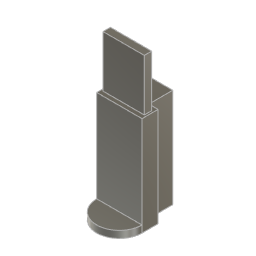
filament holder extender v1 (Autodesk Fusion 360 design; units mm, degrees)
Autodesk Fusion 360 part; units mm, degrees
note: some values were not read from the file. Set by a fixed rule: which sketch regions a step uses.
sketch "Sketch1" plane through (0, 0, 0) normal (0, 0, 1) x (1, 0, 0)
  line L0 (0, 0) -> (12.6, 0)
  line L1 (12.6, 0) -> (12.6, 13)
  line L2 (12.6, 13) -> (0, 13)
  line L3 (0, 13) -> (0, 0)
  line L4 (6.3, 0) -> (6.3, 25)
  line L5 (12.6, 13) -> (17.6, 13)
  line L6 (17.6, 13) -> (17.6, 19.7)
  line L7 (17.6, 19.7) -> (12.6, 19.7)
  line L8 (12.6, 19.7) -> (12.6, 13)
  line L9 (0, 19.7) -> (0, 13)
  line L10 (-5, 19.7) -> (0, 19.7)
  line L11 (-5, 13) -> (-5, 19.7)
  line L12 (0, 13) -> (-5, 13)
  line L13 (12.6, 19.7) -> (0, 19.7)
  line L14 (0, 19.7) -> (12.6, 13) construction
  line L15 (17.5, 18.35) -> (-4.9, 18.35)
  line L16 (-4.9, 18.35) -> (-4.9, 14.35)
  line L17 (-4.9, 14.35) -> (17.5, 14.35)
  line L18 (17.5, 14.35) -> (17.5, 18.35)
  line L19 (17.5, 18.35) -> (-4.9, 14.35) construction
  line L20 (-4.9, 18.35) -> (17.5, 14.35) construction
  line L21 (12.6, 20.7) -> (0, 20.7)
  line L22 (-6, 20.7) -> (0, 20.7)
  line L23 (-6, 12) -> (-6, 20.7)
  line L24 (-1, 12) -> (-6, 12)
  line L25 (-1, 12) -> (-1, -1)
  line L26 (-1, -1) -> (13.6, -1)
  line L27 (13.6, -1) -> (13.6, 12)
  line L28 (13.6, 12) -> (18.6, 12)
  line L29 (18.6, 12) -> (18.6, 20.7)
  line L30 (18.6, 20.7) -> (12.6, 20.7)
  point P0 (6.3, 16.35)
  dimension "d1" = 12.6
  dimension "d2" = 13
  dimension "d3" = 5
  dimension "d4" = 6.7
  dimension "d5" = 22.4
  dimension "d6" = 4
  dimension "d7" = 1
  constraint horizontal L0
  constraint vertical L1
  constraint horizontal L2
  constraint vertical L3
  constraint coincident L0.start L3.end
  constraint midpoint L0 L4.start
  constraint perpendicular L2 L4
  constraint horizontal L5
  constraint vertical L6
  constraint horizontal L7
  constraint vertical L8
  constraint symmetric L1.end L4 L2.end
  constraint symmetric L4 L5.end L11.start
  constraint symmetric L4 L6.end L10.start
  constraint symmetric L4 L7.end L9.start
  constraint horizontal L15
  constraint perpendicular L15 L16
  constraint parallel L15 L17
  constraint parallel L16 L18
  constraint coincident L19 P0
  constraint coincident L20 P0
  constraint midpoint L14 P0
  measures "d1" distance of L0.start L0.end
  measures "d2" distance of L0.start L2.end
  measures "d3" distance of L1.end L5.end
  measures "d4" distance of L1.end L7.end
  measures "d5" distance of L16.end L17.end
  measures "d6" distance of L15.end L16.end
extrude "Extrude1" add sketch "Sketch1" along normal blind 50 contours L0 L2 L3 L4 | L0 L1 L2 L4 | L2 L4 L9 L17 | L9 L10 L11 L12 L15 L16 L17 | L2 L4 L8 L17 | L9 L15 L16 L17 | L4 L9 L15 L17 | L5 L6 L7 L8 L15 L17 L18 | L4 L8 L15 L17 | L4 L9 L13 L15 | L8 L15 L17 L18 | L4 L8 L13 L15 | L21 L22 L23 L24 L25 L26 L27 L28 L29 L30
extrude "Extrude2" add sketch "Sketch1" against normal blind 28 contours L9 L15 L16 L17 | L4 L9 L15 L17 | L4 L8 L15 L17 | L8 L15 L17 L18
sketch "Sketch2" plane through (0, 0, 50) normal (0, 0, 1) x (-1, 0, 0)
  line L0 (1, -12) -> (1, 1)
  line L1 (1, 1) -> (-13.6, 1)
  line L2 (-13.6, 1) -> (-13.6, -12)
  line L3 (-13.6, -12) -> (-18.6, -12)
  line L4 (-18.6, -12) -> (-18.6, -20.7)
  line L5 (-18.6, -20.7) -> (6, -20.7)
  line L6 (6, -20.7) -> (6, -12)
  line L7 (6, -12) -> (1, -12)
  circle A0 centre (-6.3, -20.7) radius 12.3
  constraint midpoint L5 A0.centre
  constraint coincident L4.end A0
extrude "Extrude3" add sketch "Sketch2" along normal blind 3.8 contours L0 L2 L3 L5 L7 A0 | L0 L1 L2 A0 | L6 L7 A0 | L5 A0 | L3 L4 A0
move_body "Move1" bodies 1 to x (1, 0, 0) y (0, -1, 0) z (0, 0, -1) at (0, -2, 0)
move_body "Move2" bodies 1 to x (1, 0, 0) y (0, 1, 0) z (0, 0, 1) at (0, 0, 54)
equation "d5 = 13 mm + 4.7 mm + 4.7 mm"
